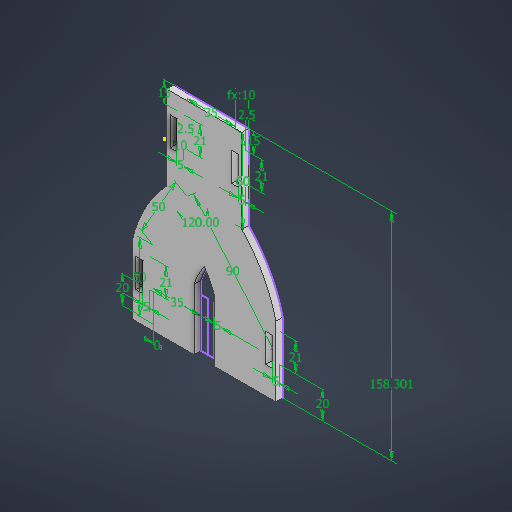
# Autodesk Inventor part: newmiddle
Saved by Autodesk Inventor 2026.2 (Build 302298000, 298)
## iProperties
Created: 2026-04-08
Part Number: newmiddle
Material: Generic
Document SubType Name: Modeling
Designer: danda
Density: 1 g/cm^3
Appearance: Default
Author: danda
Autodesk Inventor part; units mm, degrees
ref_plane "YZ Plane" through (0, 0, 0) normal (1, 0, 0) x (0, 1, 0)
ref_plane "XZ Plane" through (0, 0, 0) normal (0, 1, 0) x (-1, 0, 0)
ref_plane "XY Plane" through (0, 0, 0) normal (0, 0, 1) x (1, 0, 0)
sketch "Sketch1" plane through (0, 0, 0) normal (0, 0, 1) x (1, 0, 0)
  line L0 (51.2872, 31.5555) -> (51.2872, -28.4445)
  line L1 (16.2872, 31.5555) -> (16.2872, -28.4445)
  arc A0 (16.2872, -28.4445) -> (-8.7128, -71.7458) centre (78.6621, -93.3242) ccw
  line L2 (16.2872, -28.4445) -> (-8.7128, -71.7458) construction
  line L3 (16.2872, -28.4445) -> (66.2872, -28.4445) construction
  line L4 (-8.7128, -71.7458) -> (-8.7128, -121.7458)
  arc A1 (76.1491, -71.1938) -> (51.2872, -28.4445) centre (-11.0876, -93.3242) ccw
  line L5 (76.1491, -71.1938) -> (76.1491, -121.1332)
  line L6 (26.2872, -121.7458) -> (26.2872, -76.5352)
  arc A2 (33.7872, -61.5241) -> (26.2872, -76.5352) centre (78.6621, -93.3242) ccw
  arc A3 (41.1491, -76.1101) -> (33.7872, -61.5241) centre (-11.0876, -93.3242) ccw
  line L7 (41.1491, -76.1101) -> (41.1491, -121.1332)
  line L8 (-18.7128, -121.1332) -> (-18.7128, -70.5617)
  arc A4 (6.2872, -24.3178) -> (-18.7128, -70.5617) centre (78.6621, -93.3242) ccw
  line L9 (6.2872, -24.3178) -> (6.2872, 37.168)
  line L10 (6.2872, 37.168) -> (61.2872, 37.168)
  line L11 (61.2872, 37.168) -> (61.2872, -24.3178)
  arc A5 (86.1491, -69.9786) -> (61.2872, -24.3178) centre (-11.0876, -93.3242) ccw
  line L12 (86.1491, -69.9786) -> (86.1491, -121.1332)
  line L13 (-18.7128, -121.1332) -> (86.1491, -121.1332)
  line L14 (16.2872, 31.5555) -> (16.2872, 37.168)
  line L15 (51.2872, 31.5555) -> (51.2872, 37.168)
  line L16 (36.1491, -121.1332) -> (36.1491, -85.5895)
  line L17 (31.2872, -85.5895) -> (31.2872, -121.7458)
  line L18 (26.2872, -85.5895) -> (31.2872, -85.5895)
  line L19 (36.1491, -85.5895) -> (41.1491, -85.5895)
  line L20 (50.9283, 31.5555) -> (51.2872, 31.5555)
  line L21 (16.2872, 2.168) -> (16.2872, 22.168)
  line L22 (51.2872, 2.168) -> (51.2872, 22.168)
  line L23 (76.1491, -101.1332) -> (76.1491, -81.1332)
  line L24 (-8.7128, -81.1332) -> (-8.7128, -101.1332)
  line L25 (78.6491, -80.1332) -> (83.6491, -80.1332)
  line L26 (83.6491, -80.1332) -> (83.6491, -101.1332)
  line L27 (83.6491, -101.1332) -> (78.6491, -101.1332)
  line L28 (78.6491, -101.1332) -> (78.6491, -80.1332)
  line L29 (-16.1906, -80.1332) -> (-11.1906, -80.1332)
  line L30 (-11.1906, -80.1332) -> (-11.1906, -101.1332)
  line L31 (-11.1906, -101.1332) -> (-16.1906, -101.1332)
  line L32 (-16.1906, -101.1332) -> (-16.1906, -80.1332)
  line L33 (53.7872, 22.168) -> (58.7872, 22.168)
  line L34 (58.7872, 22.168) -> (58.7872, 1.168)
  line L35 (58.7872, 1.168) -> (53.7872, 1.168)
  line L36 (53.7872, 1.168) -> (53.7872, 22.168)
  line L37 (8.7872, 22.168) -> (13.7872, 22.168)
  line L38 (13.7872, 22.168) -> (13.7872, 1.168)
  line L39 (13.7872, 1.168) -> (8.7872, 1.168)
  line L40 (8.7872, 1.168) -> (8.7872, 22.168)
  point P0 (0, 0)
  point P1 (-8.7128, -121.1332)
  point P2 (26.2872, -121.1332)
  point P3 (36.2872, -121.7458)
  point P4 (71.2872, -121.7458)
  point P5 (31.2872, -121.1332)
  point P6 (31.2872, -121.7458)
  dimension "d0" = 35
  dimension "d1" = 60
  dimension "d2" = 50
  dimension "d3" = 120
  dimension "d4" = 90
  dimension "d5" = 50
  dimension "d6" = 35
  dimension "d7" = 10
  dimension "d12" = 5
  dimension "d16" = 10
  dimension "d22" = 158.3013
  dimension "d29" = 0
  dimension "d30" = 5
  dimension "d31" = 21
  dimension "d32" = 5
  dimension "d33" = 21
  dimension "d34" = 5
  dimension "d35" = 21
  dimension "d36" = 5
  dimension "d37" = 21
  dimension "d38" = 2.5
  dimension "d39" = 15
  dimension "d40" = 2.5
  dimension "d41" = 15
  dimension "d42" = 20
  dimension "d43" = 20
  constraints: 82 end point, 13 point on line, 12 point on circle, 9 perpendicular, 8 parallel, 7 horizontal, 6 centre point, 2 vertical, 1 equal length, 5 other
  measures "d0" distance of L1.start L0.start
  measures "d1" distance of L0.start L0.end
  measures "d2" distance of L1.end L2.end
  measures "d3" angle of L2 L3
  measures "d4" radius of A0
  measures "d5" distance of L2.end L4.end
  measures "d6" distance between parallel lines of L4 L6
  measures "d7" distance between parallel lines of L1 L9
  measures "d12" distance between parallel lines of L7 L16
  measures "d16" distance between parallel lines of L11 L0
  measures "d22" distance between parallel lines of L13 L10
  measures "d29" distance between parallel lines of L4 L24
  measures "d30" distance of L26.end L27.end
  measures "d31" distance of L25.end L26.end
  measures "d32" distance of L30.end L31.end
  measures "d33" distance of L29.end L30.end
  measures "d34" distance of L34.end L35.end
  measures "d35" distance of L33.end L34.end
  measures "d36" distance of L38.end L39.end
  measures "d37" distance of L37.end L38.end
  measures "d38" distance between parallel lines of L1 L38
  measures "d39" distance between parallel lines of L10 L37
  measures "d40" distance between parallel lines of L11 L34
  measures "d41" distance between parallel lines of L10 L33
  measures "d42" distance between parallel lines of L13 L31
  measures "d43" distance between parallel lines of L13 L27
extrude "Extrusion1" add sketch "Sketch1" along normal blind 5 contours L15 L10 L11 A5 L12 L13 L5 A1 L0 | L0 A1 L5 L13 L7 A3 A2 L6 L4 A0 L1 L14 L10 L15 | L14 L1 A0 L4 L13 L8 A4 L9 L10
equation "\"d16\" = d7"
body "Solid1"
